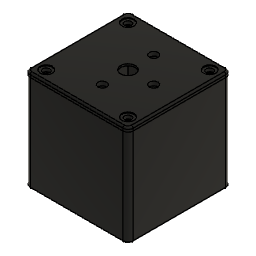
Receiver_Box (Autodesk Fusion 360 design; units mm, degrees)
Autodesk Fusion 360 part; units mm, degrees
sketch "Sketch1" plane through (0, 0, 0) normal (0, 0, 1) x (1, 0, 0)
  line L0 (30, -30) -> (-30, -30)
  line L1 (-30, -30) -> (-30, 30)
  line L2 (-30, 30) -> (30, 30)
  line L3 (30, 30) -> (30, -30)
  line L4 (30, -30) -> (-30, 30) construction
  line L5 (-30, -30) -> (30, 30) construction
  dimension "d1" = 60
  dimension "d2" = 60
  constraint horizontal L0
  constraint perpendicular L0 L1
  constraint parallel L0 L2
  constraint parallel L1 L3
  constraint coincident L4 origin
  constraint coincident L5 origin
  measures "d1" distance of L1.end L2.end
  measures "d2" distance of L0.end L1.end
extrude "Extrude1" add sketch "Sketch1" along normal blind 2.4 makes body 1
sketch "Sketch2" plane through (0, 0, 2.4) normal (0, 0, 1) x (-1, 0, 0)
  line L0 (-30, -30) -> (30, -30)
  line L1 (30, -30) -> (30, 30)
  line L2 (30, 30) -> (-30, 30)
  line L3 (-30, 30) -> (-30, -30)
  line L4 (-27.6, -27.6) -> (27.6, -27.6)
  line L5 (27.6, -27.6) -> (27.6, 27.6)
  line L6 (27.6, 27.6) -> (-27.6, 27.6)
  line L7 (-27.6, 27.6) -> (-27.6, -27.6)
  line L8 (-27.6, -27.6) -> (27.6, 27.6) construction
  line L9 (27.6, -27.6) -> (-27.6, 27.6) construction
  dimension "d7" = 2.4
  dimension "d8" = 2.4
  constraint horizontal L4
  constraint perpendicular L4 L5
  constraint parallel L4 L6
  constraint parallel L5 L7
  constraint coincident L8 origin
  constraint coincident L9 origin
  measures "d7" distance of L0 L4
  measures "d8" distance of L1 L5
extrude "Extrude2" add sketch "Sketch2" along normal blind 54 bodies 1
sketch "Sketch3" plane through (0, 0, 56.4) normal (0, 0, 1) x (-1, 0, 0)
  line L0 (-27.6, -27.6) -> (-27.6, 27.6)
  line L1 (-27.6, 27.6) -> (27.6, 27.6)
  line L2 (27.6, 27.6) -> (27.6, -27.6)
  line L3 (27.6, -27.6) -> (-27.6, -27.6)
  line L4 (-30, 30) -> (-30, -30)
  line L5 (-30, -30) -> (30, -30)
  line L6 (30, -30) -> (30, 30)
  line L7 (30, 30) -> (-30, 30)
  line L8 (-30, 30) -> (30, 30)
  line L9 (30, 30) -> (30, -30)
  line L10 (30, -30) -> (-30, -30)
  line L11 (-30, -30) -> (-30, 30)
  constraint horizontal L8
  constraint vertical L9
  constraint horizontal L10
  constraint vertical L11
  constraint coincident L5.end L6.start
  constraint coincident L4.start L7.end
extrude "Extrude3" add sketch "Sketch3" along normal blind 2.4 separate body contours L0 L1 L2 L3 | L4 L5 L6 L7 L8 L9 L10 L11 makes body 2
sketch "Sketch4" plane through (-27.6, 0, 0) normal (1, 0, 0) x (0, 1, 0)
  line L0 (-27.6, 2.4) -> (27.6, 2.4)
  line L1 (27.6, 2.4) -> (27.6, 56.4)
  line L2 (27.6, 56.4) -> (-27.6, 56.4)
  line L3 (-27.6, 56.4) -> (-27.6, 2.4)
  line L4 (-27.6, 56.4) -> (-17.6, 56.4)
  line L5 (-17.6, 56.4) -> (-17.6, 52.4)
  line L6 (-17.6, 52.4) -> (-27.6, 52.4)
  line L7 (-27.6, 52.4) -> (-27.6, 56.4)
  line L8 (27.6, 56.4) -> (17.6, 56.4)
  line L9 (17.6, 56.4) -> (17.6, 52.4)
  line L10 (17.6, 52.4) -> (27.6, 52.4)
  line L11 (27.6, 52.4) -> (27.6, 56.4)
  dimension "d13" = 10
  dimension "d14" = 10
  dimension "d22" = 4
  dimension "d23" = 4
  constraint horizontal L4
  constraint vertical L5
  constraint horizontal L6
  constraint vertical L7
  constraint coincident L2.end L3.start
  constraint horizontal L8
  constraint vertical L9
  constraint horizontal L10
  constraint vertical L11
  constraint coincident L1.end L2.start
  measures "d13" distance of L5 L7
  measures "d14" distance of L9 L11
  measures "d22" distance of L4.end L5.end
  measures "d23" distance of L8.end L9.end
extrude "Extrude4" add sketch "Sketch4" along normal blind 10 contours L2 L3 L4 L5 L6 L7 | L1 L2 L8 L9 L10 L11 bodies 1
mirror "Mirror1" about plane through (0, 0, 0) normal (1, 0, 0) of "Extrude4"
sketch "Sketch8" plane through (0, 0, 56.4) normal (0, 0, 1) x (-1, 0, 0)
  line L0 (-27.6, -17.6) -> (-27.6, 17.6)
  line L1 (-27.6, 17.6) -> (-17.6, 17.6)
  line L2 (-17.6, 17.6) -> (-17.6, 27.6)
  line L3 (-17.6, 27.6) -> (17.6, 27.6)
  line L4 (17.6, 27.6) -> (17.6, 17.6)
  line L5 (17.6, 17.6) -> (27.6, 17.6)
  line L6 (27.6, 17.6) -> (27.6, -17.6)
  line L7 (27.6, -17.6) -> (17.6, -17.6)
  line L8 (17.6, -17.6) -> (17.6, -27.6)
  line L9 (17.6, -27.6) -> (-17.6, -27.6)
  line L10 (-17.6, -27.6) -> (-17.6, -17.6)
  line L11 (-17.6, -17.6) -> (-27.6, -17.6)
  line L12 (-30, 30) -> (-30, -30)
  line L13 (-30, -30) -> (30, -30)
  line L14 (30, -30) -> (30, 30)
  line L15 (30, 30) -> (-30, 30)
  circle A0 centre (-23.8, 23.8) radius 1.25
  circle A1 centre (23.8, 23.8) radius 1.25
  dimension "d27" = 2.5
  dimension "d28" = 6.2
  dimension "d29" = 6.2
  dimension "d30" = 2.5
  dimension "d31" = 6.2
  dimension "d32" = 6.2
  measures "d27" diameter of A0
  measures "d28" distance of L2 A0.centre
  measures "d29" distance of L1 A0.centre
  measures "d30" diameter of A1
  measures "d31" distance of L15 A1.centre
  measures "d32" distance of L14 A1.centre
extrude "Extrude5" cut sketch "Sketch8" against normal blind 4 contours A0 | A1 bodies 1
mirror "Mirror2" about plane through (0, 0, 0) normal (0, 1, 0) of "Extrude5"
sketch "Sketch9" plane through (0, 0, 58.8) normal (0, 0, 1) x (-1, 0, 0)
  line L0 (-30, -30) -> (30, -30)
  line L1 (30, -30) -> (30, 30)
  line L2 (30, 30) -> (-30, 30)
  line L3 (-30, 30) -> (-30, -30)
  circle A0 centre (-23.8, 23.8) radius 2
  circle A1 centre (23.8, 23.8) radius 2
  dimension "d37" = 4
  dimension "d38" = 6.2
  dimension "d39" = 6.2
  dimension "d40" = 4
  dimension "d41" = 6.2
  dimension "d42" = 6.2
  measures "d37" diameter of A0
  measures "d38" distance of L2 A0.centre
  measures "d39" distance of L3 A0.centre
  measures "d40" diameter of A1
  measures "d41" distance of L2 A1.centre
  measures "d42" distance of L1 A1.centre
extrude "Extrude6" cut sketch "Sketch9" against normal blind 2.4 contours A0 | A1 bodies 2
mirror "Mirror3" about plane through (0, 0, 0) normal (0, 1, 0) of "Extrude6"
sketch "Sketch10" plane through (0, 0, 58.8) normal (0, 0, 1) x (-1, 0, 0)
  circle A0 centre (-23.8, -23.8) radius 2
  circle A1 centre (23.8, -23.8) radius 2
  circle A2 centre (-23.8, 23.8) radius 2
  circle A3 centre (23.8, 23.8) radius 2
  line L0 (-30, -30) -> (30, -30)
  line L1 (30, -30) -> (30, 30)
  line L2 (30, 30) -> (-30, 30)
  line L3 (-30, 30) -> (-30, -30)
  circle A4 centre (-23.8, 23.8) radius 3.5
  circle A5 centre (-23.8, -23.8) radius 3.5
  dimension "d47" = 7
  dimension "d49" = 7
  constraint concentric A2 A4
  constraint concentric A0 A5
  measures "d47" diameter of A4
  measures "d49" diameter of A5
extrude "Extrude7" cut sketch "Sketch10" against normal blind 0.5 contours A4 | A5 bodies 2
mirror "Mirror4" about plane through (0, 0, 0) normal (1, 0, 0) of "Extrude7"
fillet "Fillet1" radius 5 4 edges at (-17.6, -17.6, 54.4) (-17.6, 17.6, 54.4) (17.6, 17.6, 54.4) (17.6, -17.6, 54.4) on bodies 1
fillet "Fillet2" radius 3 4 edges at (30, 30, 28.2) (30, -30, 28.2) (-30, -30, 28.2) (-30, 30, 28.2) on bodies 1
fillet "Fillet4" radius 3 4 edges at (30, 30, 57.6) (30, -30, 57.6) (-30, -30, 57.6) (-30, 30, 57.6) on bodies 2
sketch "Sketch11" plane through (0, 0, 58.8) normal (0, 0, 1) x (-1, 0, 0)
  circle A0 centre (23.8, 23.8) radius 3.5
  circle A1 centre (23.8, -23.8) radius 3.5
  circle A2 centre (-23.8, 23.8) radius 3.5
  circle A3 centre (-23.8, -23.8) radius 3.5
  arc A4 (27, -30) -> (30, -27) centre (27, -27) ccw
  line L0 (30, -27) -> (30, 27)
  arc A5 (30, 27) -> (27, 30) centre (27, 27) ccw
  line L1 (27, 30) -> (-27, 30)
  arc A6 (-27, 30) -> (-30, 27) centre (-27, 27) ccw
  line L2 (-30, 27) -> (-30, -27)
  arc A7 (-30, -27) -> (-27, -30) centre (-27, -27) ccw
  line L3 (-27, -30) -> (27, -30)
  circle A8 centre (0, 0) radius 6.1
  circle A9 centre (-15, 0) radius 2.5
  circle A10 centre (0, 15) radius 2.5
  circle A11 centre (15, 0) radius 2.5
  circle A12 centre (0, 0) radius 4.25
  dimension "d63" = 12.2
  dimension "d64" = 5
  dimension "d65" = 15
  dimension "d66" = 15
  dimension "d67" = 30
  dimension "d68" = 5
  dimension "d69" = 15
  dimension "d70" = 5
  dimension "d71" = 15
  dimension "d90" = 8.5
  constraint coincident A8.centre A12.centre
  constraint concentric A8 A12
  measures "d63" diameter of A8
  measures "d64" diameter of A9
  measures "d65" distance of A8.centre A9.centre
  measures "d66" distance of L2 A9.centre
  measures "d67" distance of L1 A9.centre
  measures "d68" diameter of A10
  measures "d69" distance of A8.centre A10.centre
  measures "d70" diameter of A11
  measures "d71" distance of A8.centre A11.centre
  measures "d90" diameter of A12
extrude "Extrude8" cut sketch "Sketch11" against normal blind 2.4 contours A9 | A10 | A11 | A12 bodies 2
sketch "Sketch12" plane through (0, 30, 0) normal (0, 1, 0) x (-1, 0, 0)
  line L0 (27, 0) -> (27, 56.4)
  line L1 (27, 56.4) -> (-27, 56.4)
  line L2 (-27, 56.4) -> (-27, 0)
  line L3 (-27, 0) -> (27, 0)
  line L4 (-3.75, 18.7) -> (3.75, 18.7)
  line L5 (3.75, 18.7) -> (3.75, 16.85)
  line L6 (3.75, 16.85) -> (3.25, 16.5)
  line L7 (3.25, 16.5) -> (3.25, 15)
  line L8 (3.25, 15) -> (-3.25, 15)
  line L9 (-3.25, 15) -> (-3.25, 16.5)
  line L10 (-3.25, 16.5) -> (-3.75, 16.85)
  line L11 (-3.75, 16.85) -> (-3.75, 18.7)
  constraint horizontal L4
  constraint perpendicular L4 L5
  constraint perpendicular L4 L7
  constraint perpendicular L7 L8
  constraint perpendicular L4 L9
  constraint perpendicular L4 L11
sketch "Sketch13" plane through (0, 27.6, 0) normal (0, 1, 0) x (-1, 0, 0)
  line L0 (27, 0) -> (27, 56.4)
  line L1 (27, 56.4) -> (-27, 56.4)
  line L2 (-27, 56.4) -> (-27, 0)
  line L3 (-27, 0) -> (27, 0)
  line L4 (3.75, 19.81) -> (-3.75, 19.81)
  line L5 (-3.75, 19.81) -> (-3.75, 17.96)
  line L6 (-3.75, 17.96) -> (-3.25, 17.61)
  line L7 (-3.25, 17.61) -> (-3.25, 16.11)
  line L8 (-3.25, 16.11) -> (3.25, 16.11)
  line L9 (3.25, 16.11) -> (3.25, 17.61)
  line L10 (3.25, 17.61) -> (3.75, 17.96)
  line L11 (3.75, 17.96) -> (3.75, 19.81)
  line L12 (-3.45, 19.51) -> (3.45, 19.51)
  line L13 (3.45, 19.51) -> (3.45, 18.1162)
  line L14 (3.45, 18.1162) -> (2.95, 17.7662)
  line L15 (2.95, 17.7662) -> (2.95, 16.41)
  line L16 (2.95, 16.41) -> (-2.95, 16.41)
  line L17 (-2.95, 16.41) -> (-2.95, 17.7662)
  line L18 (-2.95, 17.7662) -> (-3.45, 18.1162)
  line L19 (-3.45, 18.1162) -> (-3.45, 19.51)
  line L20 (-4.15, 17.7517) -> (-3.65, 17.4017)
  line L21 (-3.65, 17.4017) -> (-3.65, 15.71)
  line L22 (-3.65, 15.71) -> (3.65, 15.71)
  line L23 (3.65, 15.71) -> (3.65, 17.4017)
  line L24 (3.65, 17.4017) -> (4.15, 17.7517)
  line L25 (4.15, 17.7517) -> (4.15, 20.21)
  line L26 (4.15, 20.21) -> (-4.15, 20.21)
  line L27 (-4.15, 20.21) -> (-4.15, 17.7517)
  line L28 (8.95, 16.11) -> (-8.95, 16.11)
  line L29 (-8.95, 16.11) -> (-8.95, 14.51)
  line L30 (-8.95, 14.51) -> (8.95, 14.51)
  line L31 (8.95, 14.51) -> (8.95, 16.11)
  line L32 (-9.35, 14.11) -> (9.35, 14.11)
  line L33 (9.35, 14.11) -> (9.35, 16.51)
  line L34 (9.35, 16.51) -> (-9.35, 16.51)
  line L35 (-9.35, 16.51) -> (-9.35, 14.11)
  line L36 (-27.6, 52.4) -> (-17.6, 52.4)
  line L37 (-17.6, 52.4) -> (-17.6, 56.4)
  line L38 (-17.6, 56.4) -> (17.6, 56.4)
  line L39 (17.6, 56.4) -> (17.6, 52.4)
  line L40 (17.6, 52.4) -> (27.6, 52.4)
  line L41 (27.6, 52.4) -> (27.6, 2.4)
  line L42 (27.6, 2.4) -> (-27.6, 2.4)
  line L43 (-27.6, 2.4) -> (-27.6, 52.4)
  dimension "d79" = 0.4
  dimension "d80" = 0.4
extrude "Extrude10" cut sketch "Sketch13" along normal through all contours L4 L5 L6 L7 L9 L10 L11 L12 L13 L14 L15 L17 L18 L19 L34 | L4 L5 L6 L7 L9 L10 L11 L20 L21 L23 L24 L25 L26 L27 L34 | L9 L23 L28 L34 | L7 L8 L9 L15 L16 L17 L28 L34 | L7 L21 L28 L34 | L8 L21 L22 L23 L28 | L12 L13 L14 L15 L17 L18 L19 L34 | L15 L16 L17 L34 bodies 1
extrude "Extrude11" cut sketch "Sketch13" along normal blind 1 contours L9 L23 L28 L34 | L7 L8 L9 L15 L16 L17 L28 L34 | L7 L21 L28 L34 | L8 L21 L22 L23 L28 | L21 L23 L28 L29 L30 L31 L32 L33 L34 L35 | L15 L16 L17 L34 | L21 L22 L23 L28 L29 L30 L31 bodies 1
sketch "Sketch14" plane through (0, 0, 56.4) normal (0, 0, -1) x (1, 0, 0)
  circle A0 centre (15, 0) radius 2.5
  circle A1 centre (0, 15) radius 2.5
  circle A2 centre (-15, 0) radius 2.5
  arc A3 (-30, -27) -> (-27, -30) centre (-27, -27) ccw
  line L0 (-27, -30) -> (27, -30)
  arc A4 (27, -30) -> (30, -27) centre (27, -27) ccw
  line L1 (30, -27) -> (30, 27)
  arc A5 (30, 27) -> (27, 30) centre (27, 27) ccw
  line L2 (27, 30) -> (-27, 30)
  arc A6 (-27, 30) -> (-30, 27) centre (-27, 27) ccw
  line L3 (-30, 27) -> (-30, -27)
  circle A7 centre (23.8, -23.8) radius 2
  circle A8 centre (-23.8, -23.8) radius 2
  circle A9 centre (23.8, 23.8) radius 2
  circle A10 centre (-23.8, 23.8) radius 2
  line L4 (-17.489, -1.566) -> (-17.489, 0)
  circle A11 centre (-14.989, 0) radius 2.5
  line L5 (-17.489, 0) -> (-17.489, 1.566)
  arc A12 (-17.489, -1.566) -> (-17.489, 1.566) centre (-14.989, 0) ccw
  line L6 (-2.489, 13.434) -> (-2.489, 15)
  circle A13 centre (0.011, 15) radius 2.5
  line L7 (-2.489, 15) -> (-2.489, 16.566)
  arc A14 (-2.489, 13.434) -> (-2.489, 16.566) centre (0.011, 15) ccw
  line L8 (16.612, -2.535) -> (15.0459, -2.535)
  circle A15 centre (15.0459, -0.035) radius 2.5
  line L9 (15.0459, -2.535) -> (13.4799, -2.535)
  arc A16 (16.612, -2.535) -> (13.4799, -2.535) centre (15.0459, -0.035) ccw
  circle A17 centre (-14.989, 0) radius 2.65
  circle A18 centre (0.011, 15) radius 2.65
  circle A19 centre (15.0459, -0.035) radius 2.65
  circle A20 centre (0, 0) radius 4.25
  dimension "d85" = 0.15
  dimension "d86" = 0.15
  dimension "d87" = 0.15
extrude "Extrude12" add sketch "Sketch14" along normal blind 5.8 contours L8 L9 A16 A19 | L6 L7 A14 A18 | L4 L5 A12 A17 bodies 2
sketch "Sketch15" plane through (0, 0, 56.4) normal (0, 0, -1) x (1, 0, 0)
  line L0 (16.612, -2.535) -> (15.9248, -2.535)
  arc A0 (15.9248, -2.535) -> (14.167, -2.535) centre (15.0459, -0.035) ccw
  line L1 (14.167, -2.535) -> (13.4799, -2.535)
  arc A1 (16.612, -2.535) -> (13.4799, -2.535) centre (15.0459, -0.035) ccw
  line L2 (-2.489, 13.434) -> (-2.489, 14.1211)
  arc A2 (-2.489, 14.1211) -> (-2.489, 15.8789) centre (0.011, 15) ccw
  line L3 (-2.489, 15.8789) -> (-2.489, 16.566)
  arc A3 (-2.489, 13.434) -> (-2.489, 16.566) centre (0.011, 15) ccw
  line L4 (-17.489, -1.566) -> (-17.489, -0.8789)
  arc A4 (-17.489, -0.8789) -> (-17.489, 0.8789) centre (-14.989, 0) ccw
  line L5 (-17.489, 0.8789) -> (-17.489, 1.566)
  arc A5 (-17.489, -1.566) -> (-17.489, 1.566) centre (-14.989, 0) ccw
  circle A6 centre (0, 15) radius 2.5
  circle A7 centre (0, 0) radius 4.25
  circle A8 centre (15, 0) radius 2.5
  circle A9 centre (-15, 0) radius 2.5
  arc A10 (-30, -27) -> (-27, -30) centre (-27, -27) ccw
  line L6 (-27, -30) -> (27, -30)
  arc A11 (27, -30) -> (30, -27) centre (27, -27) ccw
  line L7 (30, -27) -> (30, 27)
  arc A12 (30, 27) -> (27, 30) centre (27, 27) ccw
  line L8 (27, 30) -> (-27, 30)
  arc A13 (-27, 30) -> (-30, 27) centre (-27, 27) ccw
  line L9 (-30, 27) -> (-30, -27)
  circle A14 centre (23.8, -23.8) radius 2
  circle A15 centre (-23.8, -23.8) radius 2
  circle A16 centre (23.8, 23.8) radius 2
  circle A17 centre (-23.8, 23.8) radius 2
  circle A18 centre (0, 0) radius 6.1
extrude "Extrude13" cut sketch "Sketch15" against normal blind 1.4 contours A18 bodies 2
sketch "Sketch16" plane through (0, 0, 56.4) normal (0, 0, -1) x (1, 0, 0)
  circle A0 centre (0, 0) radius 6.1
  line L0 (16.612, -2.535) -> (15.9248, -2.535)
  arc A1 (15.9248, -2.535) -> (14.167, -2.535) centre (15.0459, -0.035) ccw
  line L1 (14.167, -2.535) -> (13.4799, -2.535)
  arc A2 (16.612, -2.535) -> (13.4799, -2.535) centre (15.0459, -0.035) ccw
  line L2 (-2.489, 13.434) -> (-2.489, 14.1211)
  arc A3 (-2.489, 14.1211) -> (-2.489, 15.8789) centre (0.011, 15) ccw
  line L3 (-2.489, 15.8789) -> (-2.489, 16.566)
  arc A4 (-2.489, 13.434) -> (-2.489, 16.566) centre (0.011, 15) ccw
  line L4 (-17.489, -1.566) -> (-17.489, -0.8789)
  arc A5 (-17.489, -0.8789) -> (-17.489, 0.8789) centre (-14.989, 0) ccw
  line L5 (-17.489, 0.8789) -> (-17.489, 1.566)
  arc A6 (-17.489, -1.566) -> (-17.489, 1.566) centre (-14.989, 0) ccw
  circle A7 centre (0, 15) radius 2.5
  circle A8 centre (15, 0) radius 2.5
  circle A9 centre (-15, 0) radius 2.5
  arc A10 (-30, -27) -> (-27, -30) centre (-27, -27) ccw
  line L6 (-27, -30) -> (27, -30)
  arc A11 (27, -30) -> (30, -27) centre (27, -27) ccw
  line L7 (30, -27) -> (30, 27)
  arc A12 (30, 27) -> (27, 30) centre (27, 27) ccw
  line L8 (27, 30) -> (-27, 30)
  arc A13 (-27, 30) -> (-30, 27) centre (-27, 27) ccw
  line L9 (-30, 27) -> (-30, -27)
  circle A14 centre (23.8, -23.8) radius 2
  circle A15 centre (-23.8, -23.8) radius 2
  circle A16 centre (23.8, 23.8) radius 2
  circle A17 centre (-23.8, 23.8) radius 2
  circle A18 centre (-0.0073, -10.0111) radius 1.75
  circle A19 centre (-0.0073, -10.0111) radius 0.9
  dimension "d93" = -0.85
extrude "Extrude14" add sketch "Sketch16" along normal blind 7.6 contours A18 bodies 2
sketch "Sketch17" plane through (27.6, 0, 0) normal (-1, 0, 0) x (0, -1, 0)
  line L0 (-17.6, 52.4) -> (-27.6, 52.4)
  line L1 (-27.6, 52.4) -> (-27.6, 2.4)
  line L2 (-27.6, 2.4) -> (27.6, 2.4)
  line L3 (27.6, 2.4) -> (27.6, 52.4)
  line L4 (27.6, 52.4) -> (17.6, 52.4)
  line L5 (17.6, 52.4) -> (17.6, 56.4)
  line L6 (17.6, 56.4) -> (-17.6, 56.4)
  line L7 (-17.6, 56.4) -> (-17.6, 52.4)
  line L8 (-7.668, 25.85) -> (-10.068, 25.85)
  line L9 (-10.068, 25.85) -> (-10.068, 28.25)
  line L10 (-10.068, 28.25) -> (-7.668, 28.25)
  line L11 (-7.668, 28.25) -> (-7.668, 25.85)
  line L12 (-7.668, 25.85) -> (-10.068, 28.25) construction
  line L13 (-10.068, 25.85) -> (-7.668, 28.25) construction
  line L14 (-17.368, 25.85) -> (-19.768, 25.85)
  line L15 (-19.768, 25.85) -> (-19.768, 28.25)
  line L16 (-19.768, 28.25) -> (-17.368, 28.25)
  line L17 (-17.368, 28.25) -> (-17.368, 25.85)
  line L18 (-17.368, 25.85) -> (-19.768, 28.25) construction
  line L19 (-19.768, 25.85) -> (-17.368, 28.25) construction
  line L20 (-26.718, 23.25) -> (-26.718, 24.5)
  line L21 (-0.718, 23.25) -> (-0.718, 24.5)
  point P0 (-8.868, 27.05)
  point P1 (-18.568, 27.05)
  dimension "d100" = 2.4
  dimension "d101" = 2.4
  dimension "d102" = 2.4
  dimension "d103" = 2.4
  dimension "d104" = 6.95
  dimension "d105" = 6.95
  constraint horizontal L8
  constraint perpendicular L8 L9
  constraint parallel L8 L10
  constraint parallel L9 L11
  constraint coincident L12 P0
  constraint coincident L13 P0
  constraint horizontal L14
  constraint perpendicular L14 L15
  constraint parallel L14 L16
  constraint parallel L15 L17
  constraint coincident L18 P1
  constraint coincident L19 P1
  measures "d100" distance of L9.end L10.end
  measures "d101" distance of L15.end L16.end
  measures "d102" distance of L14.end L15.end
  measures "d103" distance of L8.start L10.end
  measures "d104" distance of L15 L20
  measures "d105" distance of L11 L21
extrude "Extrude15" add sketch "Sketch17" along normal blind 21.9375 contours L8 L9 L10 L11 | L14 L15 L16 L17 bodies 1
sketch "Sketch18" plane through (0, 0, 28.25) normal (0, 0, 1) x (-1, 0, 0)
  line L0 (-27.6, -10.068) -> (-5.6625, -10.068)
  line L1 (-5.6625, -10.068) -> (-5.6625, -7.668)
  line L2 (-5.6625, -7.668) -> (-27.6, -7.668)
  line L3 (-8.0625, -7.668) -> (-5.6625, -7.668)
  line L4 (-5.6625, -7.668) -> (-5.6625, -10.068)
  line L5 (-5.6625, -10.068) -> (-8.0625, -10.068)
  line L6 (-8.0625, -10.068) -> (-8.0625, -7.668)
  line L7 (-8.0625, -7.668) -> (-5.6625, -10.068) construction
  line L8 (-5.6625, -7.668) -> (-8.0625, -10.068) construction
  line L9 (-8.0625, -17.368) -> (-5.6625, -17.368)
  line L10 (-5.6625, -17.368) -> (-5.6625, -19.768)
  line L11 (-5.6625, -19.768) -> (-8.0625, -19.768)
  line L12 (-8.0625, -19.768) -> (-8.0625, -17.368)
  line L13 (-8.0625, -17.368) -> (-5.6625, -19.768) construction
  line L14 (-5.6625, -17.368) -> (-8.0625, -19.768) construction
  line L15 (-27.6, -7.668) -> (-27.6, -10.068)
  point P0 (-6.8625, -8.868)
  point P1 (-6.8625, -18.568)
  point P2 (-5.6625, -19.768)
  dimension "d108" = 2.4
  dimension "d109" = 2.4
  dimension "d110" = 2.4
  dimension "d111" = 2.4
  constraint horizontal L3
  constraint perpendicular L3 L4
  constraint parallel L3 L5
  constraint parallel L4 L6
  constraint coincident L7 P0
  constraint coincident L8 P0
  constraint coincident L0.end L1.start
  constraint horizontal L9
  constraint perpendicular L9 L10
  constraint parallel L9 L11
  constraint parallel L10 L12
  constraint coincident L13 P1
  constraint coincident L14 P1
  constraint coincident P2 L10.end
  measures "d108" distance of L0.end L5.end
  measures "d109" distance of L1.end L0.end
  measures "d110" distance of P2 L11.end
  measures "d111" distance of L9.end P2
extrude "Extrude16" add sketch "Sketch18" along normal blind 2.4 contours L0 L1 L2 L3 L4 L5 L6 | L9 L10 L11 L12 bodies 1
sketch "Sketch19" plane through (0, 0, 2.4) normal (0, 0, 1) x (-1, 0, 0)
  line L0 (-27.6, -27.6) -> (27.6, -27.6)
  line L1 (27.6, -27.6) -> (27.6, 27.6)
  line L2 (27.6, 27.6) -> (-27.6, 27.6)
  line L3 (-27.6, 27.6) -> (-27.6, -27.6)
  line L4 (-21.833, -7.668) -> (-19.433, -7.668)
  line L5 (-19.433, -7.668) -> (-19.433, -10.068)
  line L6 (-19.433, -10.068) -> (-21.833, -10.068)
  line L7 (-21.833, -10.068) -> (-21.833, -7.668)
  line L8 (-21.833, -7.668) -> (-19.433, -10.068) construction
  line L9 (-19.433, -7.668) -> (-21.833, -10.068) construction
  line L10 (-21.833, -17.368) -> (-19.433, -17.368)
  line L11 (-19.433, -17.368) -> (-19.433, -19.768)
  line L12 (-19.433, -19.768) -> (-21.833, -19.768)
  line L13 (-21.833, -19.768) -> (-21.833, -17.368)
  line L14 (-21.833, -17.368) -> (-19.433, -19.768) construction
  line L15 (-19.433, -17.368) -> (-21.833, -19.768) construction
  line L16 (-27.6, -19.768) -> (-8.0625, -19.768)
  line L17 (-27.6, -10.068) -> (-8.0625, -10.068)
  point P0 (-20.633, -8.868)
  point P1 (-20.633, -18.568)
  dimension "d114" = 2.4
  dimension "d115" = 2.4
  dimension "d116" = 2.4
  dimension "d117" = 2.4
  dimension "d118" = 6.967
  dimension "d119" = 6.967
  constraint horizontal L4
  constraint perpendicular L4 L5
  constraint parallel L4 L6
  constraint parallel L5 L7
  constraint coincident L8 P0
  constraint coincident L9 P0
  constraint horizontal L10
  constraint perpendicular L10 L11
  constraint parallel L10 L12
  constraint parallel L11 L13
  constraint coincident L14 P1
  constraint coincident L15 P1
  constraint coincident L11.end L16
  constraint coincident L5.end L17
  measures "d114" distance of L5.end L6.end
  measures "d115" distance of L4.end L5.end
  measures "d116" distance of L11.end L12.end
  measures "d117" distance of L10.end L11.end
  measures "d118" distance of L3 P1
  measures "d119" distance of L3 P0
extrude "Extrude17" add sketch "Sketch19" along normal blind 23.5 contours L4 L5 L6 L7 L17 | L10 L11 L12 L13 L16 bodies 1
sketch "Sketch20" plane through (-27.6, 0, 0) normal (1, 0, 0) x (0, 1, 0)
  line L0 (17.6, 52.4) -> (17.6, 56.4)
  line L1 (17.6, 56.4) -> (-17.6, 56.4)
  line L2 (-17.6, 56.4) -> (-17.6, 52.4)
  line L3 (-17.6, 52.4) -> (-27.6, 52.4)
  line L4 (-27.6, 52.4) -> (-27.6, 2.4)
  line L5 (-27.6, 2.4) -> (27.6, 2.4)
  line L6 (27.6, 2.4) -> (27.6, 52.4)
  line L7 (27.6, 52.4) -> (17.6, 52.4)
  line L8 (-4.8, 32.3) -> (4.8, 32.3)
  line L9 (4.8, 32.3) -> (4.8, 29.9)
  line L10 (4.8, 29.9) -> (-4.8, 29.9)
  line L11 (-4.8, 29.9) -> (-4.8, 32.3)
  line L12 (-19.3127, 11.9) -> (27.4873, 11.9)
  line L13 (0, 56.4) -> (0, 11.9)
  line L14 (4.8, 46) -> (-4.8, 46)
  line L15 (-4.8, 46) -> (-4.8, 48.4)
  line L16 (-4.8, 48.4) -> (4.8, 48.4)
  line L17 (4.8, 48.4) -> (4.8, 46)
  line L18 (4.8, 46) -> (-4.8, 48.4) construction
  line L19 (-4.8, 46) -> (4.8, 48.4) construction
  line L20 (21.6, 41.8) -> (19.2, 41.8)
  line L21 (19.2, 41.8) -> (19.2, 51.4)
  line L22 (19.2, 51.4) -> (21.6, 51.4)
  line L23 (21.6, 51.4) -> (21.6, 41.8)
  line L24 (21.6, 41.8) -> (19.2, 51.4) construction
  line L25 (19.2, 41.8) -> (21.6, 51.4) construction
  point P0 (0, 47.2)
  point P1 (20.4, 46.6)
  dimension "d122" = 9.6
  dimension "d123" = 2.4
  dimension "d124" = 18
  dimension "d125" = 4.8
  dimension "d126" = 9.6
  dimension "d127" = 2.4
  dimension "d128" = 8
  dimension "d194" = 2.4
  dimension "d195" = 9.6
  dimension "d196" = 1
  dimension "d197" = 6
  constraint horizontal L8
  constraint vertical L9
  constraint horizontal L10
  constraint vertical L11
  constraint midpoint L1 L13.start
  constraint coincident L12 L13.end
  constraint perpendicular L12 L13
  constraint horizontal L14
  constraint perpendicular L14 L15
  constraint parallel L14 L16
  constraint parallel L15 L17
  constraint coincident L18 P0
  constraint coincident L19 P0
  constraint coincident L13 P0
  constraint horizontal L20
  constraint perpendicular L20 L21
  constraint parallel L20 L22
  constraint parallel L21 L23
  constraint coincident L24 P1
  constraint coincident L25 P1
  measures "d122" distance of L8.start L8.end
  measures "d123" distance of L8.start L10.end
  measures "d124" distance of L10 L12
  measures "d125" distance of L9 L13
  measures "d126" distance of L15.end L16.end
  measures "d127" distance of L14.end L15.end
  measures "d128" distance of L1 L16
  measures "d194" distance of L21.end L22.end
  measures "d195" distance of L20.end L21.end
  measures "d196" distance of L7 L22
  measures "d197" distance of L6 L23
fillet "Fillet7" radius 0.5 28 edges at (5.6625, 7.668, 28.25) (5.6625, 10.068, 28.25) (5.6625, 17.368, 28.25) (5.6625, 19.768, 28.25) (6.8625, 7.668, 30.65) (6.8625, 10.068, 30.65) (12.5477, 7.668, 25.85) (6.8625, 17.368, 30.65) (12.5477, 17.368, 25.85) (24.7165, 7.668, 25.85) (19.433, 7.668, 14.125) (19.433, 10.068, 14.125) (21.833, 7.668, 14.125) (21.833, 10.068, 14.125) (24.7165, 10.068, 25.85) (12.5477, 10.068, 25.85) (5.6625, 8.868, 25.85) (5.6625, 8.868, 30.65) (6.8625, 19.768, 30.65) (24.7165, 17.368, 25.85) (19.433, 17.368, 14.125) (21.833, 17.368, 14.125) (19.433, 19.768, 14.125) (21.833, 19.768, 14.125) (24.7165, 19.768, 25.85) (12.5477, 19.768, 25.85) (5.6625, 18.568, 25.85) (5.6625, 18.568, 30.65) on bodies 1
sketch "Sketch24" plane through (0, 27.6, 0) normal (0, -1, 0) x (1, 0, 0)
  line L0 (-9.35, 16.51) -> (-3.65, 16.51)
  line L1 (-3.65, 16.51) -> (-3.65, 17.4017)
  line L2 (-3.65, 17.4017) -> (-4.15, 17.7517)
  line L3 (-4.15, 17.7517) -> (-4.15, 20.21)
  line L4 (-4.15, 20.21) -> (4.15, 20.21)
  line L5 (4.15, 20.21) -> (4.15, 17.7517)
  line L6 (4.15, 17.7517) -> (3.65, 17.4017)
  line L7 (3.65, 17.4017) -> (3.65, 16.51)
  line L8 (3.65, 16.51) -> (9.35, 16.51)
  line L9 (9.35, 16.51) -> (9.35, 14.11)
  line L10 (9.35, 14.11) -> (-9.35, 14.11)
  line L11 (-9.35, 14.11) -> (-9.35, 16.51)
  line L12 (27.6, 52.4) -> (17.6, 52.4)
  line L13 (17.6, 52.4) -> (17.6, 56.4)
  line L14 (17.6, 56.4) -> (-17.6, 56.4)
  line L15 (-17.6, 56.4) -> (-17.6, 52.4)
  line L16 (-17.6, 52.4) -> (-27.6, 52.4)
  line L17 (-27.6, 52.4) -> (-27.6, 2.4)
  line L18 (-27.6, 2.4) -> (27.6, 2.4)
  line L19 (27.6, 2.4) -> (27.6, 52.4)
  line L20 (21.6, 41.8) -> (19.2, 41.8)
  line L21 (19.2, 41.8) -> (19.2, 51.4)
  line L22 (19.2, 51.4) -> (21.6, 51.4)
  line L23 (21.6, 51.4) -> (21.6, 41.8)
  line L24 (21.6, 41.8) -> (19.2, 51.4) construction
  line L25 (19.2, 41.8) -> (21.6, 51.4) construction
  point P0 (20.4, 46.6)
  dimension "d178" = 2.4
  dimension "d179" = 9.6
  dimension "d180" = 6
  dimension "d181" = 1
  constraint horizontal L20
  constraint perpendicular L20 L21
  constraint parallel L20 L22
  constraint parallel L21 L23
  constraint coincident L24 P0
  constraint coincident L25 P0
  measures "d178" distance of L21.end L22.end
  measures "d179" distance of L20.end L21.end
  measures "d180" distance of L19 L23
  measures "d181" distance of L12 L22
sketch "Sketch28" plane through (0, 27.6, 0) normal (0, -1, 0) x (1, 0, 0)
  line L0 (-9.35, 16.51) -> (-3.65, 16.51)
  line L1 (-3.65, 16.51) -> (-3.65, 17.4017)
  line L2 (-3.65, 17.4017) -> (-4.15, 17.7517)
  line L3 (-4.15, 17.7517) -> (-4.15, 20.21)
  line L4 (-4.15, 20.21) -> (4.15, 20.21)
  line L5 (4.15, 20.21) -> (4.15, 17.7517)
  line L6 (4.15, 17.7517) -> (3.65, 17.4017)
  line L7 (3.65, 17.4017) -> (3.65, 16.51)
  line L8 (3.65, 16.51) -> (9.35, 16.51)
  line L9 (9.35, 16.51) -> (9.35, 14.11)
  line L10 (9.35, 14.11) -> (-9.35, 14.11)
  line L11 (-9.35, 14.11) -> (-9.35, 16.51)
  line L12 (27.6, 52.4) -> (17.6, 52.4)
  line L13 (17.6, 52.4) -> (17.6, 56.4)
  line L14 (17.6, 56.4) -> (-17.6, 56.4)
  line L15 (-17.6, 56.4) -> (-17.6, 52.4)
  line L16 (-17.6, 52.4) -> (-27.6, 52.4)
  line L17 (-27.6, 52.4) -> (-27.6, 2.4)
  line L18 (-27.6, 2.4) -> (27.6, 2.4)
  line L19 (27.6, 2.4) -> (27.6, 52.4)
  line L20 (-4.0784, 37.8398) -> (4.0816, 37.8398)
  arc A0 (4.3816, 37.5398) -> (4.0816, 37.8398) centre (4.0816, 37.5398) ccw
  line L21 (4.3816, 37.5398) -> (4.3816, 27.2398)
  arc A1 (-4.0784, 37.8398) -> (-4.3784, 37.5398) centre (-4.0784, 37.5398) ccw
  line L22 (-4.3784, 27.2398) -> (-4.3784, 37.5398)
  line L23 (4.0816, 27.0398) -> (-4.0784, 27.0398)
  arc A2 (-4.3784, 27.2398) -> (-4.1784, 27.0398) centre (-4.1784, 27.2398) ccw
  line L24 (-4.0784, 27.0398) -> (-4.1784, 27.0398)
  arc A3 (4.1816, 27.0398) -> (4.3816, 27.2398) centre (4.1816, 27.2398) ccw
  line L25 (4.1816, 27.0398) -> (4.0816, 27.0398)
  circle A4 centre (0.0016, 33.3598) radius 3
  line L26 (4.1816, 26.6398) -> (4.0816, 26.6398)
  line L27 (4.0816, 26.6398) -> (-4.0784, 26.6398)
  line L28 (-4.0784, 26.6398) -> (-4.1784, 26.6398)
  arc A5 (-4.7784, 27.2398) -> (-4.1784, 26.6398) centre (-4.1784, 27.2398) ccw
  line L29 (-4.7784, 27.2398) -> (-4.7784, 37.5398)
  arc A6 (-4.0784, 38.2398) -> (-4.7784, 37.5398) centre (-4.0784, 37.5398) ccw
  line L30 (-4.0784, 38.2398) -> (4.0816, 38.2398)
  arc A7 (4.7816, 37.5398) -> (4.0816, 38.2398) centre (4.0816, 37.5398) ccw
  line L31 (4.7816, 37.5398) -> (4.7816, 27.2398)
  arc A8 (4.1816, 26.6398) -> (4.7816, 27.2398) centre (4.1816, 27.2398) ccw
  circle A9 centre (0.0016, 33.3598) radius 3.4
  dimension "d228" = -0.4
  dimension "d229" = 0.4
extrude "Extrude29" cut sketch "Sketch28" against normal through all contours A4 | A9 bodies 1
extrude "Extrude30" cut sketch "Sketch28" against normal blind 1.2 contours L20 A0 L21 A1 L22 L23 A2 L24 A3 L25 | L26 L27 L28 A5 L29 A6 L30 A7 L31 A8 bodies 1
fillet "Fillet13" radius 1 16 edges at (-29.1213, -29.1213, 0) (-30, 0, 0) (-29.1213, 29.1213, 0) (0, 30, 0) (29.1213, 29.1213, 0) (30, 0, 0) (29.1213, -29.1213, 0) (0, -30, 0) (29.1213, -29.1213, 58.8) (30, 0, 58.8) (29.1213, 29.1213, 58.8) (0, 30, 58.8) (-29.1213, 29.1213, 58.8) (-30, 0, 58.8) (-29.1213, -29.1213, 58.8) (0, -30, 58.8) on bodies 1 2
move_body "Move1" bodies 1 2 to x (0, 1, 0) y (-1, 0, 0) z (0, 0, 1) at (0, 0, 0)
equation "d3 = boxWidth"
equation "d7 = boxWidth"
equation "d8 = boxWidth"
equation "d11 = boxWidth"
equation "boxWidth = 2.4 mm"
equation "d23 = d22"
equation "d27 = boxScrewHoleWidth"
equation "d30 = boxScrewHoleWidth"
equation "d43 = -boxWidth"
equation "d47 = boxSanfren"
equation "boxSanfren = 7 mm"
equation "d49 = boxSanfren"
equation "boxSanfrenDepth = 0.5 mm"
equation "d51 = -boxSanfrenDepth"
equation "d69 = d65"
equation "d72 = -boxWidth"
equation "boxScrewHoleWidth = 2.5 mm"
equation "d106 = 18.1375 mm + 3.8 mm"
equation "d120 = 18.5 mm + 5 mm"
equation "d163 = 1 mm"
equation "d176 = d163"
equation "d177 = 6 mm"
equation "d180 = d177"
equation "d181 = d176"
named bodies: "Case", "Cap"
